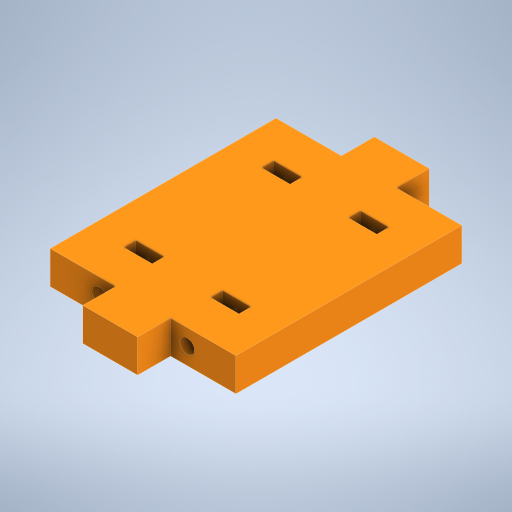
# Autodesk Inventor part: bridge_hands1
Saved by Autodesk Inventor 2024 (Build 280153000, 153)
## iProperties
Created: 2024-09-08
Part Number: bridge_hands1
Material: PMMA 플라스틱
Document SubType Name: Modeling
Designer: jmha0
Density: 1.188 g/cm^3
Appearance: 주황색
Author: jmha0
Autodesk Inventor part; units mm, degrees
ref_plane "YZ Plane" through (0, 0, 0) normal (1, 0, 0) x (0, 1, 0)
ref_plane "XZ Plane" through (0, 0, 0) normal (0, 1, 0) x (-1, 0, 0)
ref_plane "XY Plane" through (0, 0, 0) normal (0, 0, 1) x (1, 0, 0)
sketch "스케치8" plane through (0, 0, 0) normal (0, 0, 1) x (1, 0, 0)
  circle A0 centre (12.1807, -22.6311) radius 1.2
  arc A1 (9.2807, -22.6311) -> (14.3807, -22.6311) centre (11.8307, -22.1236) ccw
  circle A2 centre (14.5238, -16.9742) radius 1.2
  circle A3 centre (20.1807, -14.6311) radius 1.2
  circle A4 centre (25.8375, -16.9742) radius 1.2
  circle A5 centre (28.1807, -22.6311) radius 1.2
  arc A6 (25.9807, -22.6311) -> (31.0807, -22.6311) centre (28.5307, -22.1236) ccw
  line L0 (9.2807, -22.6311) -> (31.0807, -22.6311)
  line L1 (9.2807, -2.6311) -> (9.2807, -22.6311)
  line L2 (31.0807, -22.6311) -> (31.0807, -2.6311)
  circle A7 centre (20.1807, -22.6311) radius 5.8
  line L3 (9.2807, -2.6311) -> (39.0379, -2.6311) construction
  line L4 (31.0807, -2.6311) -> (31.0807, 12.3689)
  line L5 (31.0807, 12.3689) -> (9.2807, 12.3689)
  line L6 (9.2807, 12.3689) -> (9.2807, -2.6311)
  line L7 (9.2807, 12.3689) -> (9.2807, 12.3689)
  line L8 (31.0807, 12.3689) -> (31.0807, 12.3689)
  line L9 (31.0807, 12.3689) -> (46.4956, 27.7838)
  arc A8 (46.4956, 27.7838) -> (9.2807, 12.3689) centre (31.0807, 12.3689) ccw
  arc A9 (15.2617, -2.6311) -> (15.6657, -3.046) centre (31.0807, 12.3689) ccw
  line L10 (15.1807, 15.3689) -> (25.1807, 15.3689)
  line L11 (25.1807, 15.3689) -> (25.1807, 9.3689)
  line L12 (25.1807, 9.3689) -> (15.1807, 9.3689)
  line L13 (15.1807, 9.3689) -> (15.1807, 15.3689)
  line L14 (15.1807, 15.3689) -> (25.1807, 9.3689) construction
  line L15 (25.1807, 15.3689) -> (15.1807, 9.3689) construction
  circle A10 centre (12.1807, 12.3689) radius 1.35
  circle A11 centre (28.1807, 12.3689) radius 1.35
  line L16 (9.2807, -2.6311) -> (31.0807, -2.6311)
  circle A12 centre (9.2807, 12.3689) radius 21.8
  line L17 (9.2807, 4.8689) -> (31.0807, 4.8689)
  line L18 (31.0807, 4.8689) -> (31.0807, 19.8689)
  line L19 (31.0807, 19.8689) -> (9.2807, 19.8689)
  line L20 (9.2807, 19.8689) -> (9.2807, 4.8689)
  line L21 (9.2807, 4.8689) -> (31.0807, 19.8689) construction
  line L22 (31.0807, 4.8689) -> (9.2807, 19.8689) construction
  line L23 (31.0807, 15.3689) -> (9.2807, 15.3689)
  line L24 (9.2807, 15.3689) -> (9.2807, 9.3689)
  line L25 (9.2807, 9.3689) -> (31.0807, 9.3689)
  line L26 (31.0807, 9.3689) -> (31.0807, 15.3689)
  line L27 (31.0807, 15.3689) -> (9.2807, 9.3689) construction
  line L28 (9.2807, 15.3689) -> (31.0807, 9.3689) construction
  point P0 (0, 0)
  point P1 (-60.3663, -40.6069)
  point P2 (20.1807, -22.6311)
  point P3 (20.1807, -22.6311)
  point P4 (14.3807, -22.6311)
  point P5 (14.3807, -22.6311)
  point P6 (9.2807, 17.3689)
  point P7 (25.0996, -2.6311)
  point P8 (9.2807, -9.4311)
  point P9 (20.1807, 12.3689)
  point P10 (29.7499, 19.8689)
  point P11 (10.6114, 19.8689)
  point P12 (30.8733, 15.3689)
  point P13 (9.4881, 15.3689)
  dimension "d31" = 2.6
  dimension "d32" = 2.6
  dimension "d33" = 20
  dimension "d34" = 15
  dimension "d35" = 0
  dimension "d36" = 0
  dimension "d38" = 135
  dimension "d39" = 10
  dimension "d40" = 6
  dimension "d44" = 2.7
  dimension "d45" = 2.7
  dimension "d48" = 15
  constraints: 58 end point, 12 centre point, 10 point on circle, 8 parallel, 7 midpoint, 4 horizontal, 4 perpendicular, 4 point on line, 2 coincident, 2 vertical, 1 collinear, 3 other
  measures "d31" radius of A1
  measures "d32" radius of A6
  measures "d33" distance of L2.end L0.end
  measures "d34" distance of L4.end L2.end
  measures "d35" distance of L5.end L7.end
  measures "d36" distance of L4.end L8.end
  measures "d38" angle of L9 L5
  measures "d39" distance of L11.end L12.end
  measures "d40" distance of L10.end L11.end
  measures "d44" diameter of A10
  measures "d45" diameter of A11
  measures "d48" distance of L18.end L17.end
extrude "돌출8" add sketch "스케치8" along normal blind 41.1 contours L6 L5 A10 L13 L25 | A12 L25 L11 L5 A11 | L5 A11 L11 L23 A12 | L4 L25 A12 | L23 L13 L5 A10 A8 | L13 L5 L11 L12 | A11 L5 | L5 A11 | L10 L11 L5 L13 | A10 L5 | L5 A10
sketch "스케치9" plane through (0, 0, 41.1) normal (0, 0, 1) x (1, 0, 0)
  line L0 (30.8733, 15.3689) -> (9.4881, 15.3689) projected
  line L1 (30.8733, 15.3689) -> (9.4881, 15.3689) projected
  arc A0 (9.4881, 15.3689) -> (9.2807, 12.3689) centre (31.0807, 12.3689) ccw projected
  arc A1 (9.4881, 15.3689) -> (9.2807, 12.3689) centre (31.0807, 12.3689) ccw projected
  line L2 (9.2807, 12.3689) -> (9.2807, 9.3689) projected
  line L3 (9.2807, 12.3689) -> (9.2807, 9.3689) projected
  line L4 (9.2807, 9.3689) -> (31.0807, 9.3689) projected
  line L5 (9.2807, 9.3689) -> (31.0807, 9.3689) projected
  line L6 (31.0807, 9.3689) -> (31.0807, 12.3689) projected
  line L7 (31.0807, 9.3689) -> (31.0807, 12.3689) projected
  arc A2 (31.0807, 12.3689) -> (30.8733, 15.3689) centre (9.2807, 12.3689) ccw projected
  arc A3 (31.0807, 12.3689) -> (30.8733, 15.3689) centre (9.2807, 12.3689) ccw projected
  line L8 (30.8733, 15.3689) -> (9.4881, 15.3689) projected
  arc A4 (31.0807, 12.3689) -> (30.8733, 15.3689) centre (9.2807, 12.3689) ccw projected
  line L9 (31.0807, 9.3689) -> (31.0807, 12.3689) projected
  line L10 (9.2807, 9.3689) -> (31.0807, 9.3689) projected
  line L11 (9.2807, 12.3689) -> (9.2807, 9.3689) projected
  arc A5 (9.4881, 15.3689) -> (9.2807, 12.3689) centre (31.0807, 12.3689) ccw projected
  line L12 (30.8733, 15.3689) -> (9.4881, 15.3689) projected
  arc A6 (9.4881, 15.3689) -> (9.2807, 12.3689) centre (31.0807, 12.3689) ccw projected
  line L13 (9.2807, 12.3689) -> (9.2807, 9.3689) projected
  line L14 (9.2807, 9.3689) -> (31.0807, 9.3689) projected
  line L15 (31.0807, 9.3689) -> (31.0807, 12.3689) projected
  arc A7 (31.0807, 12.3689) -> (30.8733, 15.3689) centre (9.2807, 12.3689) ccw projected
  line L16 (30.8733, 15.3689) -> (9.4881, 15.3689) projected
  line L17 (30.8733, 15.3689) -> (9.4881, 15.3689) projected
  arc A8 (9.4881, 15.3689) -> (9.2807, 12.3689) centre (31.0807, 12.3689) ccw projected
  arc A9 (9.4881, 15.3689) -> (9.2807, 12.3689) centre (31.0807, 12.3689) ccw projected
  line L18 (9.2807, 12.3689) -> (9.2807, 9.3689) projected
  line L19 (9.2807, 12.3689) -> (9.2807, 9.3689) projected
  line L20 (9.2807, 9.3689) -> (31.0807, 9.3689) projected
  line L21 (9.2807, 9.3689) -> (31.0807, 9.3689) projected
  line L22 (31.0807, 9.3689) -> (31.0807, 12.3689) projected
  line L23 (31.0807, 9.3689) -> (31.0807, 12.3689) projected
  arc A10 (31.0807, 12.3689) -> (30.8733, 15.3689) centre (9.2807, 12.3689) ccw projected
  arc A11 (31.0807, 12.3689) -> (30.8733, 15.3689) centre (9.2807, 12.3689) ccw projected
  circle A12 centre (36.2473, 1.0351) radius 1.2
  arc A13 (33.3473, 1.0351) -> (38.4473, 1.0351) centre (35.8973, 1.5425) ccw
  circle A14 centre (38.5905, 6.6919) radius 1.2
  circle A15 centre (44.2473, 9.0351) radius 1.2
  circle A16 centre (49.9042, 6.6919) radius 1.2
  circle A17 centre (52.2473, 1.0351) radius 1.2
  arc A18 (50.0473, 1.0351) -> (55.1473, 1.0351) centre (52.5973, 1.5425) ccw
  line L24 (33.3473, 1.0351) -> (55.1473, 1.0351)
  line L25 (33.3473, 21.0351) -> (33.3473, 1.0351)
  line L26 (55.1473, 1.0351) -> (55.1473, 21.0351)
  circle A19 centre (44.2473, 1.0351) radius 5.8
  line L27 (33.3473, 21.0351) -> (63.1045, 21.0351) construction
  line L28 (55.1473, 21.0351) -> (55.1473, 36.0351)
  line L29 (55.1473, 36.0351) -> (33.3473, 36.0351)
  line L30 (33.3473, 36.0351) -> (33.3473, 21.0351)
  line L31 (33.3473, 36.0351) -> (33.3473, 36.0351)
  line L32 (55.1473, 36.0351) -> (55.1473, 36.0351)
  line L33 (55.1473, 36.0351) -> (70.5623, 51.45)
  arc A20 (70.5623, 51.45) -> (33.3473, 36.0351) centre (55.1473, 36.0351) ccw
  arc A21 (39.3284, 21.0351) -> (39.7324, 20.6202) centre (55.1473, 36.0351) ccw
  line L34 (39.2473, 39.0351) -> (49.2473, 39.0351)
  line L35 (49.2473, 39.0351) -> (49.2473, 33.0351)
  line L36 (49.2473, 33.0351) -> (39.2473, 33.0351)
  line L37 (39.2473, 33.0351) -> (39.2473, 39.0351)
  line L38 (39.2473, 39.0351) -> (49.2473, 33.0351) construction
  line L39 (49.2473, 39.0351) -> (39.2473, 33.0351) construction
  circle A22 centre (36.2473, 36.0351) radius 1.35
  circle A23 centre (52.2473, 36.0351) radius 1.35
  line L40 (33.3473, 21.0351) -> (55.1473, 21.0351)
  circle A24 centre (33.3473, 36.0351) radius 21.8
  line L41 (33.3473, 28.5351) -> (55.1473, 28.5351)
  line L42 (55.1473, 28.5351) -> (55.1473, 43.5351)
  line L43 (55.1473, 43.5351) -> (33.3473, 43.5351)
  line L44 (33.3473, 43.5351) -> (33.3473, 28.5351)
  line L45 (33.3473, 28.5351) -> (55.1473, 43.5351) construction
  line L46 (55.1473, 28.5351) -> (33.3473, 43.5351) construction
  line L47 (55.1473, 39.0351) -> (33.3473, 39.0351)
  line L48 (33.3473, 39.0351) -> (33.3473, 33.0351)
  line L49 (33.3473, 33.0351) -> (55.1473, 33.0351)
  line L50 (55.1473, 33.0351) -> (55.1473, 39.0351)
  line L51 (55.1473, 39.0351) -> (33.3473, 33.0351) construction
  line L52 (33.3473, 39.0351) -> (55.1473, 33.0351) construction
  line L53 (15.1807, 15.3689) -> (25.1807, 15.3689)
  line L54 (25.1807, 15.3689) -> (25.1807, 9.3689)
  line L55 (25.1807, 9.3689) -> (15.1807, 9.3689)
  line L56 (15.1807, 9.3689) -> (15.1807, 15.3689)
  line L57 (15.1807, 15.3689) -> (25.1807, 9.3689) construction
  line L58 (25.1807, 15.3689) -> (15.1807, 9.3689) construction
  line L59 (15.1807, 12.3689) -> (12.1807, 12.3689)
  circle A25 centre (12.1807, 12.3689) radius 1.35
  line L60 (25.1807, 12.3689) -> (28.1807, 12.3689)
  circle A26 centre (28.1807, 12.3689) radius 1.35
  point P0 (0, 0)
  point P1 (24.0667, 23.6662)
  point P2 (-36.2996, -16.9407)
  point P3 (44.2473, 1.0351)
  point P4 (44.2473, 1.0351)
  point P5 (38.4473, 1.0351)
  point P6 (38.4473, 1.0351)
  point P7 (33.3473, 41.0351)
  point P8 (49.1663, 21.0351)
  point P9 (33.3473, 14.2351)
  point P10 (44.2473, 36.0351)
  point P11 (53.8166, 43.5351)
  point P12 (34.6781, 43.5351)
  point P13 (54.9399, 39.0351)
  point P14 (33.5547, 39.0351)
  point P15 (20.1807, 12.3689)
  dimension "d49" = 2.6
  dimension "d50" = 2.6
  dimension "d51" = 20
  dimension "d52" = 15
  dimension "d53" = 0
  dimension "d54" = 0
  dimension "d55" = 135
  dimension "d56" = 10
  dimension "d57" = 6
  dimension "d58" = 2.7
  dimension "d59" = 2.7
  dimension "d60" = 15
  dimension "d61" = 10
  dimension "d62" = 5.9
  dimension "d64" = 3
  dimension "d65" = 2.7
  dimension "d66" = 3
  dimension "d67" = 2.7
  constraints: 74 end point, 14 centre point, 11 midpoint, 10 parallel, 10 point on circle, 7 horizontal, 5 perpendicular, 5 point on line, 4 coincident, 2 vertical, 1 collinear, 1 horizontal alignment, 2 other
  measures "d49" radius of A13
  measures "d50" radius of A18
  measures "d51" distance of L26.end L24.end
  measures "d52" distance of L28.end L26.end
  measures "d53" distance of L29.end L31.end
  measures "d54" distance of L28.end L32.end
  measures "d55" angle of L33 L29
  measures "d56" distance of L35.end L36.end
  measures "d57" distance of L34.end L35.end
  measures "d58" diameter of A22
  measures "d59" diameter of A23
  measures "d60" distance of L42.end L41.end
  measures "d61" distance of L54.end L55.end
  measures "d62" distance of L55.end L2.end
  measures "d64" distance of L59.start L59.end
  measures "d65" diameter of A25
  measures "d66" distance of L60.start L60.end
  measures "d67" diameter of A26
extrude "돌출9" cut sketch "스케치9" against normal blind 16 contours A26 | A25
sketch "스케치10" plane through (0, 0, 41.1) normal (0, 0, 1) x (1, 0, 0)
  circle A0 centre (12.1807, 12.3689) radius 1.35 projected
  circle A1 centre (28.1807, 12.3689) radius 1.35 projected
  line L0 (30.8733, 15.3689) -> (9.4881, 15.3689) projected
  arc A2 (9.4881, 15.3689) -> (9.2807, 12.3689) centre (31.0807, 12.3689) ccw projected
  line L1 (9.2807, 12.3689) -> (9.2807, 9.3689) projected
  line L2 (9.2807, 9.3689) -> (31.0807, 9.3689) projected
  line L3 (31.0807, 9.3689) -> (31.0807, 12.3689) projected
  arc A3 (31.0807, 12.3689) -> (30.8733, 15.3689) centre (9.2807, 12.3689) ccw projected
  line L4 (15.1807, 15.3689) -> (25.1807, 15.3689)
  line L5 (25.1807, 15.3689) -> (25.1807, 9.3689)
  line L6 (25.1807, 9.3689) -> (15.1807, 9.3689)
  line L7 (15.1807, 9.3689) -> (15.1807, 15.3689)
  line L8 (15.1807, 15.3689) -> (25.1807, 9.3689) construction
  line L9 (25.1807, 15.3689) -> (15.1807, 9.3689) construction
  point P0 (0, 0)
  point P1 (20.1807, 12.3689)
  dimension "d70" = 10
  constraints: 12 end point, 2 midpoint, 2 parallel, 1 horizontal, 1 perpendicular, 1 point on line
  measures "d70" distance of L5.end L6.end
extrude "돌출10" add sketch "스케치10" along normal blind 6 contours L5 L2 L7 L0
sketch "스케치11" plane through (0, 0, 0) normal (0, 0, -1) x (-1, 0, 0)
  line L0 (-30.8733, 15.3689) -> (-9.4881, 15.3689) projected
  arc A0 (-30.8733, 15.3689) -> (-31.0807, 12.3689) centre (-9.2807, 12.3689) ccw projected
  line L1 (-31.0807, 9.3689) -> (-31.0807, 12.3689) projected
  line L2 (-9.2807, 9.3689) -> (-31.0807, 9.3689) projected
  line L3 (-9.2807, 12.3689) -> (-9.2807, 9.3689) projected
  arc A1 (-9.2807, 12.3689) -> (-9.4881, 15.3689) centre (-31.0807, 12.3689) ccw projected
  line L4 (-25.1807, 15.3689) -> (-25.1807, 9.3689) projected
  line L5 (-15.1807, 9.3689) -> (-15.1807, 15.3689) projected
  point P0 (0, 0)
extrude "돌출11" add sketch "스케치11" along normal blind 6 contours L0 L5 L2 L4
sketch "스케치12" plane through (0, 0, 0) normal (0, 0, -1) x (-1, 0, 0)
  circle A0 centre (-28.1807, 12.3689) radius 1.35 projected
  circle A1 centre (-12.1807, 12.3689) radius 1.35 projected
  point P0 (0, 0)
extrude "돌출12" cut sketch "스케치12" against normal blind 16
sketch "스케치13" plane through (9.4881, 15.3689, 41.1) normal (0, 1, 0) x (1, 0, 0)
  line L0 (17.3426, 41.1) -> (20.0426, 41.1) projected
  line L1 (17.3426, 25.1) -> (20.0426, 25.1) projected
  line L2 (21.3852, 0) -> (15.6926, 0) projected
  line L3 (15.6926, 0) -> (21.5926, 0) projected
  line L4 (15.6926, 0) -> (21.5926, 0) projected
  line L5 (21.5926, 0) -> (21.3852, 0) projected
  line L6 (21.3852, 0) -> (15.6926, 0) projected
  line L7 (20.0426, 0) -> (17.3426, 0) projected
  line L8 (15.6926, 0) -> (15.6926, -6) projected
  line L9 (15.6926, 0) -> (15.6926, -6) projected
  line L10 (15.6926, 0) -> (15.6926, -6) projected
  line L11 (15.6926, 0) -> (15.6926, -6) projected
  line L12 (4.0426, 16) -> (1.3426, 16) projected
  line L13 (4.0426, 16) -> (1.3426, 16) projected
  line L14 (4.0426, 16) -> (1.3426, 16) projected
  line L15 (4.0426, 0) -> (1.3426, 0) projected
  line L16 (5.6926, 0) -> (5.6926, -6) projected
  line L17 (5.6926, -6) -> (15.6926, -6) projected
  line L18 (15.6926, -6) -> (5.6926, -6) projected
  line L19 (5.6926, 0) -> (5.6926, -6) projected
  line L20 (5.6926, 0) -> (5.6926, -6) projected
  line L21 (1.3426, 25.1) -> (4.0426, 25.1) projected
  line L22 (21.5926, 41.1) -> (21.5926, 0) projected
  line L23 (21.3852, 41.1) -> (21.3852, 0) projected
  line L24 (21.5926, 41.1) -> (21.3852, 41.1) projected
  line L25 (21.3852, 41.1) -> (21.3852, 0) projected
  line L26 (21.5926, 0) -> (21.3852, 0) projected
  line L27 (21.5926, 41.1) -> (21.5926, 0) projected
  line L28 (21.5926, 41.1) -> (21.5926, 0) projected
  line L29 (21.5926, 41.1) -> (21.5926, 0) projected
  line L30 (21.5926, 41.1) -> (21.5926, 0) projected
  line L31 (21.3852, 41.1) -> (15.6926, 41.1) projected
  line L32 (15.6926, 41.1) -> (15.6926, 47.1) projected
  line L33 (5.6926, 47.1) -> (15.6926, 47.1) projected
  line L34 (5.6926, 41.1) -> (5.6926, 47.1) projected
  line L35 (5.6926, 41.1) -> (0, 41.1) projected
  line L36 (0, 41.1) -> (0, 0) projected
  line L37 (5.6926, 0) -> (0, 0) projected
  line L38 (5.6926, 0) -> (5.6926, -6) projected
  line L39 (15.6926, -6) -> (5.6926, -6) projected
  line L40 (15.6926, 0) -> (15.6926, -6) projected
  line L41 (21.3852, 0) -> (15.6926, 0) projected
  line L42 (21.3852, 41.1) -> (21.3852, 0) projected
  line L43 (-0.2074, 41.1) -> (5.6926, 41.1) projected
  line L44 (5.6926, 41.1) -> (5.6926, 47.1) projected
  line L45 (15.6926, 47.1) -> (5.6926, 47.1) projected
  line L46 (15.6926, 41.1) -> (15.6926, 47.1) projected
  line L47 (15.6926, 41.1) -> (21.5926, 41.1) projected
  line L48 (21.5926, 41.1) -> (21.5926, 0) projected
  line L49 (15.6926, 0) -> (21.5926, 0) projected
  line L50 (15.6926, 0) -> (15.6926, -6) projected
  line L51 (5.6926, -6) -> (15.6926, -6) projected
  line L52 (5.6926, 0) -> (5.6926, -6) projected
  line L53 (-0.2074, 0) -> (5.6926, 0) projected
  line L54 (-0.2074, 41.1) -> (-0.2074, 0) projected
  line L55 (1.3426, 41.1) -> (4.0426, 41.1) projected
  line L56 (0, 41.1) -> (0, 0) projected
  line L57 (0, 41.1) -> (-0.2074, 41.1) projected
  line L58 (-0.2074, 41.1) -> (-0.2074, 0) projected
  line L59 (0, 0) -> (-0.2074, 0) projected
  line L60 (0, 41.1) -> (0, 0) projected
  line L61 (-0.2074, 41.1) -> (-0.2074, 0) projected
  line L62 (-0.2074, 41.1) -> (-0.2074, 0) projected
  line L63 (-0.2074, 41.1) -> (-0.2074, 0) projected
  line L64 (-0.2074, 41.1) -> (-0.2074, 0) projected
  line L65 (20.0426, 0) -> (17.3426, 0) projected
  line L66 (20.0426, 16) -> (17.3426, 16) projected
  line L67 (20.0426, 16) -> (17.3426, 16) projected
  line L68 (20.0426, 16) -> (17.3426, 16) projected
  line L69 (20.0426, 0) -> (17.3426, 0) projected
  line L70 (21.3852, 0) -> (21.5926, 0) projected
  line L71 (15.6926, -6) -> (5.6926, -6) projected
  line L72 (-0.2074, 0) -> (5.6926, 0) projected
  line L73 (4.0426, 0) -> (1.3426, 0) projected
  line L74 (5.6926, 0) -> (0, 0) projected
  line L75 (-0.2074, 0) -> (0, 0) projected
  line L76 (5.6926, 0) -> (0, 0) projected
  line L77 (0, 0) -> (-0.2074, 0) projected
  line L78 (-0.2074, 0) -> (5.6926, 0) projected
  line L79 (4.0426, 0) -> (1.3426, 0) projected
  line L80 (5.6926, 0) -> (5.6926, -6) projected
  line L81 (5.6926, -6) -> (15.6926, -6) projected
  line L82 (-0.2074, 41.1) -> (5.6926, 41.1) projected
  line L83 (21.3852, 41.1) -> (15.6926, 41.1) projected
  line L84 (21.3852, 41.1) -> (21.5926, 41.1) projected
  line L85 (15.6926, 41.1) -> (21.5926, 41.1) projected
  line L86 (15.6926, 47.1) -> (5.6926, 47.1) projected
  line L87 (17.3426, 25.1) -> (20.0426, 25.1) projected
  line L88 (1.3426, 25.1) -> (4.0426, 25.1) projected
  line L89 (17.3426, 25.1) -> (20.0426, 25.1) projected
  line L90 (17.3426, 41.1) -> (20.0426, 41.1) projected
  line L91 (1.3426, 25.1) -> (4.0426, 25.1) projected
  line L92 (1.3426, 41.1) -> (4.0426, 41.1) projected
  line L93 (17.3426, 41.1) -> (20.0426, 41.1) projected
  line L94 (21.3852, 41.1) -> (15.6926, 41.1) projected
  line L95 (21.5926, 41.1) -> (21.3852, 41.1) projected
  line L96 (15.6926, 41.1) -> (21.5926, 41.1) projected
  line L97 (-0.2074, 41.1) -> (0, 41.1) projected
  line L98 (1.3426, 41.1) -> (4.0426, 41.1) projected
  line L99 (-0.2074, 41.1) -> (5.6926, 41.1) projected
  line L100 (0, 41.1) -> (-0.2074, 41.1) projected
  line L101 (5.6926, 41.1) -> (0, 41.1) projected
  line L102 (5.6926, 41.1) -> (0, 41.1) projected
  line L103 (5.6926, 47.1) -> (15.6926, 47.1) projected
  line L104 (5.6926, 41.1) -> (5.6926, 47.1) projected
  line L105 (5.6926, 41.1) -> (5.6926, 47.1) projected
  line L106 (5.6926, 47.1) -> (15.6926, 47.1) projected
  line L107 (15.6926, 47.1) -> (5.6926, 47.1) projected
  line L108 (5.6926, 41.1) -> (5.6926, 47.1) projected
  line L109 (5.6926, 41.1) -> (5.6926, 47.1) projected
  line L110 (15.6926, 41.1) -> (15.6926, 47.1) projected
  line L111 (15.6926, 41.1) -> (15.6926, 47.1) projected
  line L112 (15.6926, 41.1) -> (15.6926, 47.1) projected
  line L113 (15.6926, 41.1) -> (15.6926, 47.1) projected
  line L114 (17.3426, 41.1) -> (17.3426, 25.1) projected
  line L115 (20.0426, 41.1) -> (20.0426, 25.1) projected
  line L116 (4.0426, 41.1) -> (4.0426, 25.1) projected
  line L117 (1.3426, 41.1) -> (1.3426, 25.1) projected
  line L118 (4.0426, 0) -> (4.0426, 16) projected
  line L119 (1.3426, 0) -> (1.3426, 16) projected
  line L120 (17.3426, 0) -> (17.3426, 16) projected
  line L121 (20.0426, 0) -> (20.0426, 16) projected
  line L122 (0.2463, 32) -> (5.4463, 32)
  line L123 (5.4463, 32) -> (5.4463, 34.2)
  line L124 (5.4463, 34.2) -> (0.2463, 34.2)
  line L125 (0.2463, 34.2) -> (0.2463, 32)
  line L126 (0.2463, 32) -> (5.4463, 34.2) construction
  line L127 (5.4463, 32) -> (0.2463, 34.2) construction
  line L128 (16.0426, 32) -> (21.2426, 32)
  line L129 (21.2426, 32) -> (21.2426, 34.2)
  line L130 (21.2426, 34.2) -> (16.0426, 34.2)
  line L131 (16.0426, 34.2) -> (16.0426, 32)
  line L132 (16.0426, 32) -> (21.2426, 34.2) construction
  line L133 (21.2426, 32) -> (16.0426, 34.2) construction
  line L134 (16.0426, 6.9) -> (21.2426, 6.9)
  line L135 (21.2426, 6.9) -> (21.2426, 9.1)
  line L136 (21.2426, 9.1) -> (16.0426, 9.1)
  line L137 (16.0426, 9.1) -> (16.0426, 6.9)
  line L138 (16.0426, 6.9) -> (21.2426, 9.1) construction
  line L139 (21.2426, 6.9) -> (16.0426, 9.1) construction
  line L140 (0.2463, 6.9) -> (5.4463, 6.9)
  line L141 (5.4463, 6.9) -> (5.4463, 9.1)
  line L142 (5.4463, 9.1) -> (0.2463, 9.1)
  line L143 (0.2463, 9.1) -> (0.2463, 6.9)
  line L144 (0.2463, 6.9) -> (5.4463, 9.1) construction
  line L145 (5.4463, 6.9) -> (0.2463, 9.1) construction
  point P0 (-9.4881, 41.1)
  point P1 (2.8463, 33.1)
  point P2 (18.6426, 33.1)
  point P3 (18.6426, 8)
  point P4 (2.8463, 8)
  dimension "d77" = 5.2
  dimension "d78" = 2.2
  dimension "d79" = 5.2
  dimension "d80" = 2.2
  dimension "d81" = 5.2
  dimension "d82" = 2.2
  dimension "d83" = 5.2
  dimension "d84" = 2.2
  constraints: 48 end point, 8 midpoint, 8 parallel, 4 horizontal, 4 perpendicular, 11 other
  measures "d77" distance of L124.end L123.end
  measures "d78" distance of L123.end L122.end
  measures "d79" distance of L130.end L129.end
  measures "d80" distance of L129.end L128.end
  measures "d81" distance of L136.end L135.end
  measures "d82" distance of L135.end L134.end
  measures "d83" distance of L142.end L141.end
  measures "d84" distance of L141.end L140.end
extrude "돌출13" cut sketch "스케치13" against normal blind 10 contours L130 L115 L128 L114 | L114 L128 L131 L130 | L130 L129 L128 L115 | L134 L120 L136 L121 | L121 L136 L135 L134 | L134 L137 L136 L120 | L124 L123 L122 L116 | L116 L122 L117 L124 | L117 L122 L125 L124 | L140 L143 L142 L119 | L119 L142 L118 L140 | L118 L142 L141 L140
sketch "스케치14" plane through (9.2807, 9.3689, 0) normal (-1, 0, 0) x (0, 0, 1)
  line L0 (0, 6) -> (0, 3) projected
  line L1 (0, 3) -> (41.1, 3) projected
  line L2 (41.1, 6) -> (41.1, 3) projected
  line L3 (0, 6) -> (41.1, 6) projected
  line L4 (0, 3) -> (0, 0) projected
  line L5 (0, 0) -> (41.1, 0) projected
  line L6 (41.1, 3) -> (41.1, 0) projected
  line L7 (0, 3) -> (41.1, 3) projected
  line L8 (0, 0) -> (0, 6) projected
  line L9 (41.1, 0) -> (47.1, 0) projected
  line L10 (0, 6) -> (41.1, 6)
  line L11 (41.1, 6) -> (41.1, 0)
  line L12 (41.1, 0) -> (0, 0)
  line L13 (0, 0) -> (0, 6)
  point P0 (0, -9.3689)
  constraints: 8 end point, 2 parallel, 1 horizontal, 1 perpendicular
extrude "돌출14" add sketch "스케치14" along normal blind 6
sketch "스케치15" plane through (31.0807, 9.3689, 0) normal (1, 0, 0) x (0, 0, -1)
  line L0 (-32, 1.65) -> (-25.1, 1.65) projected
  line L1 (0, 0) -> (0, 3) projected
  line L2 (0, 3) -> (-41.1, 3) projected
  line L3 (-41.1, 0) -> (-41.1, 3) projected
  line L4 (0, 0) -> (-41.1, 0) projected
  line L5 (0, 3) -> (0, 6) projected
  line L6 (0, 6) -> (-41.1, 6) projected
  line L7 (-41.1, 3) -> (-41.1, 6) projected
  line L8 (0, 3) -> (-41.1, 3) projected
  point P0 (0, -9.3689)
extrude "돌출15" add sketch "스케치15" along normal blind 6
sketch "스케치16" plane through (9.4881, 15.3689, 41.1) normal (0, 1, 0) x (1, 0, 0)
  line L0 (-0.2074, 0) -> (-0.2074, 41.1) projected
  line L1 (-0.2074, 41.1) -> (-6.2074, 41.1) projected
  line L2 (-6.2074, 0) -> (-6.2074, 41.1) projected
  line L3 (-0.2074, 0) -> (-6.2074, 0) projected
  line L4 (5.4463, 34.2) -> (5.4463, 32) projected
  line L5 (5.4463, 32) -> (0.2463, 32) projected
  line L6 (0.2463, 32) -> (0.2463, 34.2) projected
  line L7 (0.2463, 34.2) -> (5.4463, 34.2) projected
  line L8 (21.2426, 9.1) -> (21.2426, 6.9) projected
  line L9 (21.2426, 6.9) -> (16.0426, 6.9) projected
  line L10 (16.0426, 6.9) -> (16.0426, 9.1) projected
  line L11 (16.0426, 9.1) -> (21.2426, 9.1) projected
  line L12 (21.2426, 34.2) -> (21.2426, 32) projected
  line L13 (21.2426, 32) -> (16.0426, 32) projected
  line L14 (16.0426, 32) -> (16.0426, 34.2) projected
  line L15 (16.0426, 34.2) -> (21.2426, 34.2) projected
  line L16 (5.4463, 9.1) -> (5.4463, 6.9) projected
  line L17 (5.4463, 6.9) -> (0.2463, 6.9) projected
  line L18 (0.2463, 6.9) -> (0.2463, 9.1) projected
  line L19 (0.2463, 9.1) -> (5.4463, 9.1) projected
  line L20 (21.3852, 41.1) -> (15.6926, 41.1) projected
  line L21 (15.6926, 41.1) -> (15.6926, 47.1) projected
  line L22 (5.6926, 47.1) -> (15.6926, 47.1) projected
  line L23 (5.6926, 41.1) -> (5.6926, 47.1) projected
  line L24 (5.6926, 41.1) -> (0, 41.1) projected
  line L25 (0, 41.1) -> (0, 0) projected
  line L26 (5.6926, 0) -> (0, 0) projected
  line L27 (5.6926, 0) -> (5.6926, -6) projected
  line L28 (15.6926, -6) -> (5.6926, -6) projected
  line L29 (15.6926, 0) -> (15.6926, -6) projected
  line L30 (21.3852, 0) -> (15.6926, 0) projected
  line L31 (21.3852, 41.1) -> (21.3852, 0) projected
  line L32 (21.5926, 41.1) -> (21.5926, 0) projected
  line L33 (21.5926, 0) -> (27.5926, 0) projected
  line L34 (27.5926, 41.1) -> (27.5926, 0) projected
  line L35 (21.5926, 41.1) -> (27.5926, 41.1) projected
  line L36 (0, 41.1) -> (-0.2074, 41.1)
  line L37 (-0.2074, 41.1) -> (-0.2074, 0)
  line L38 (-0.2074, 0) -> (0, 0)
  line L39 (0, 0) -> (0, 41.1)
  line L40 (21.3852, 0) -> (21.5926, 0)
  line L41 (21.5926, 0) -> (21.5926, 41.1)
  line L42 (21.5926, 41.1) -> (21.3852, 41.1)
  line L43 (21.3852, 41.1) -> (21.3852, 0)
  point P0 (-9.4881, 41.1)
  constraints: 16 end point, 4 parallel, 2 horizontal, 2 perpendicular
extrude "돌출16" add sketch "스케치16" against normal blind 6 contours L0 L36 L25 L38 | L31 L42 L32 L40
